Autodesk Fusion 360 part; units mm, degrees
(part 2 of 2)
sketch "Sketch1 (1)" plane through (0, 0, 0) normal (0, 0, -1) x (1, 0, 0) in component "volleyball"
  arc A0 (83.3961, -53.0936) -> (83.8923, -52.463) centre (16.2304, 0.2686) ccw
  spline S0 degree 3 poles (83.1659, -53.382) (83.2447, -53.2843) (83.3214, -53.1882) (83.3961, -53.0936) knots 0.976391 0.976391 0.976391 0.976391 1 1 1 1
  arc A1 (-51.0592, -52.9372) -> (83.1659, -53.382) centre (16.2304, 0.2686) ccw
  spline S1 degree 3 poles (-51.3776, -52.5454) (-51.2718, -52.6763) (-51.1657, -52.8069) (-51.0592, -52.9372) knots 0 0 0 0 0.021256 0.021256 0.021256 0.021256
  line L0 (-51.3776, -52.5454) -> (-52.9378, -50.6056)
  line L1 (-52.9378, -50.6056) -> (-52.8595, -50.5775)
  arc A2 (-55.8686, -46.2124) -> (-52.8595, -50.5775) centre (16.2304, 0.2686) ccw
  line L2 (-55.8686, -46.2124) -> (-55.8897, -46.22)
  line L3 (-55.8897, -46.22) -> (-57.1969, -44.238)
  spline S2 degree 3 poles (-62.1595, -34.5706) (-60.5198, -38.328) (-58.7655, -41.7837) (-57.1969, -44.238) knots 0.562392 0.562392 0.562392 0.562392 1 1 1 1
  arc A3 (-63.9062, -30.3398) -> (-62.1595, -34.5706) centre (16.2304, 0.2686) ccw
  spline S3 degree 3 poles (-67.2754, -20.0749) (-66.4965, -23.1736) (-65.2961, -26.7754) (-63.9062, -30.3398) knots 0 0 0 0 0.401537 0.401537 0.401537 0.401537
  spline S4 degree 3 poles (-68.058, -15.6752) (-68.2174, -16.4999) (-67.8619, -17.7657) (-67.2754, -20.0749) knots 0.565386 0.565386 0.565386 0.565386 1 1 1 1
  arc A4 (-69.0247, -9.2348) -> (-68.058, -15.6752) centre (16.2304, 0.2686) ccw
  spline S5 degree 3 poles (-69.6369, 4.7629) (-69.9364, -0.9646) (-69.6045, -7.9217) (-69.0247, -9.2348) knots 0 0 0 0 0.88772 0.88772 0.88772 0.88772
  spline S6 degree 3 poles (-68.8618, 11.1337) (-69.2237, 11.4542) (-69.4071, 9.4617) (-69.6369, 4.7629) knots 0.394417 0.394417 0.394417 0.394417 1 1 1 1
  arc A5 (-64.9144, 28.094) -> (-68.8618, 11.1337) centre (16.2304, 0.2686) ccw
  spline S7 degree 3 poles (-62.9742, 34.0285) (-64.2565, 31.0558) (-64.713, 29.8758) (-64.9144, 28.094) knots 0 0 0 0 0.691116 0.691116 0.691116 0.691116
  spline S8 degree 3 poles (-45.01, 60.7639) (-52.3475, 53.3421) (-58.715, 43.8962) (-62.9742, 34.0285) knots 0 0 0 0 1 1 1 1
  spline S9 degree 3 poles (-33.6664, 70.3786) (-33.9616, 70.7159) (-41.2147, 64.5592) (-45.01, 60.7639) knots 0 0 0 0 1 1 1 1
  spline S10 degree 3 poles (-33.7771, 69.9679) (-33.6841, 70.2186) (-33.6421, 70.3665) (-33.6664, 70.3786) knots 0.712651 0.712651 0.712651 0.712651 1 1 1 1
  arc A6 (-23.4578, 76.3185) -> (-33.7771, 69.9679) centre (16.2304, 0.2686) ccw
  spline S11 degree 3 poles (-18.6119, 79.1077) (-21.4959, 77.8353) (-22.4841, 77.3971) (-23.4578, 76.3185) knots 0 0 0 0 0.670505 0.670505 0.670505 0.670505
  spline S12 degree 3 poles (8.1657, 86.15) (-0.9429, 85.2222) (-10.2202, 82.7764) (-18.6119, 79.1077) knots 0 0 0 0 1 1 1 1
  spline S13 degree 3 poles (13.4592, 86.007) (13.6596, 86.7737) (12.1492, 86.5306) (8.1657, 86.15) knots 0.398323 0.398323 0.398323 0.398323 1 1 1 1
  arc A7 (21.8306, 85.8687) -> (13.4592, 86.007) centre (16.2304, 0.2686) ccw
  spline S14 degree 3 poles (25.8347, 85.9813) (23.1616, 86.2075) (21.822, 86.183) (21.8306, 85.8687) knots 0 0 0 0 0.487624 0.487624 0.487624 0.487624
  spline S15 degree 3 poles (52.2328, 78.6016) (44.3893, 82.2282) (33.4674, 85.2644) (25.8347, 85.9813) knots 0 0 0 0 1 1 1 1
  spline S16 degree 3 poles (91.8721, 41.3238) (82.7214, 57.8121) (68.7633, 70.969) (52.2328, 78.6016) knots 0 0 0 0 1 1 1 1
  spline S17 degree 3 poles (93.3059, 38.4985) (93.3902, 38.4985) (92.7577, 39.7636) (91.8721, 41.3238) knots 0 0 0 0 1 1 1 1
  spline S18 degree 3 poles (92.6292, 39.281) (93.0311, 38.7947) (93.287, 38.4985) (93.3059, 38.4985) knots 0.551981 0.551981 0.551981 0.551981 1 1 1 1
  arc A8 (101.1344, 12.5184) -> (92.6292, 39.281) centre (16.2304, 0.2686) ccw
  spline S19 degree 3 poles (102.2458, 0.5459) (102.2458, 5.3459) (101.8846, 9.2629) (101.1344, 12.5184) knots 0 0 0 0 0.689854 0.689854 0.689854 0.689854
  spline S20 degree 3 poles (98.7879, -23.4906) (100.7699, -16.9544) (102.2458, -6.7494) (102.2458, 0.5459) knots 0 0 0 0 1 1 1 1
  spline S21 degree 3 poles (97.7675, -26.3857) (97.9614, -25.9701) (98.3902, -24.7924) (98.7879, -23.4906) knots 0.142524 0.142524 0.142524 0.142524 1 1 1 1
  arc A9 (94.2462, -35.4005) -> (97.7675, -26.3857) centre (16.2304, 0.2686) ccw
  line L4 (94.2462, -35.4005) -> (94.318, -35.6776)
  line L5 (94.318, -35.6776) -> (92.5468, -39.009)
  spline S22 degree 3 poles (91.7936, -40.3388) (92.0288, -39.9459) (92.2777, -39.5051) (92.5468, -39.009) knots 0.80059 0.80059 0.80059 0.80059 1 1 1 1
  arc A10 (85.3416, -50.5487) -> (91.7936, -40.3388) centre (16.2304, 0.2686) ccw
  line L6 (85.3416, -50.5487) -> (85.4202, -50.5213)
  line L7 (85.4202, -50.5213) -> (83.8923, -52.463)
  spline S23 degree 3 poles (15.4189, -90.4979) (12.72, -90.4558) (8.9248, -90.2449) (6.9428, -90.0762) knots 0 0 0 0 1 1 1 1
  spline S24 degree 3 poles (102.6253, -27.8341) (90.354, -65.4493) (54.8473, -90.9196) (15.4189, -90.4979) knots 0 0 0 0 1 1 1 1
  spline S25 degree 3 poles (98.2397, 39.9744) (108.5291, 18.6788) (110.0472, -5.1048) (102.6253, -27.8341) knots 0 0 0 0 1 1 1 1
  spline S26 degree 3 poles (29.9252, 90.5778) (59.4438, 86.0656) (85.2093, 66.9629) (98.2397, 39.9744) knots 0 0 0 0 1 1 1 1
  spline S27 degree 3 poles (-48.0883, 64.8544) (-27.594, 85.3066) (1.5451, 94.9212) (29.9252, 90.5778) knots 0 0 0 0 1 1 1 1
  spline S28 degree 3 poles (-73.137, 17.8354) (-69.7213, 35.5888) (-61.0344, 51.9084) (-48.0883, 64.8544) knots 0 0 0 0 1 1 1 1
  spline S29 degree 3 poles (-48.0462, -63.7625) (-69.5526, -42.2982) (-78.872, -11.9784) (-73.137, 17.8354) knots 0 0 0 0 1 1 1 1
  spline S30 degree 3 poles (6.9428, -90.0762) (-13.5515, -87.9678) (-33.2869, -78.5218) (-48.0462, -63.7625) knots 0 0 0 0 1 1 1 1
  line L8 (-29.2215, 67.0521) -> (-27.2782, 62.1333)
  line L9 (16.0482, 23.5133) -> (16.9632, 18.2905)
  spline S31 degree 5 poles (-29.2215, 67.0521) (-27.2169, 67.844) (-23.1769, 69.2849) (-17.024, 71.0173) (-8.6346, 72.4691) (2.1466, 72.8543) (13.1771, 71.8135) (24.3659, 69.3547) (35.5625, 65.493) (46.5368, 60.2511) (56.9839, 53.666) (66.561, 45.8033) (74.916, 36.7693) (81.7202, 26.725) (86.6971, 15.8966) (89.658, 4.5944) (90.5182, -6.7944) (89.2793, -17.8574) (86.0193, -28.199) (80.8797, -37.4875) (74.0534, -45.4973) (65.7727, -52.1602) (56.2994, -57.5184) (45.9154, -61.6662) (34.9127, -64.694) (23.5847, -66.6367) (12.2152, -67.406) (1.0725, -66.7803) (-9.5904, -64.493) (-19.5366, -60.2966) (-28.5457, -54.0387) (-36.4147, -45.7289) (-42.9583, -35.6201) (-48.0121, -24.156) (-51.436, -11.9035) (-53.1176, 0.5089) (-52.9751, 12.4565) (-50.9619, 23.3791) (-47.0678, 32.8512) (-41.3393, 40.5784) (-33.9011, 46.3842) (-24.9773, 50.2007) (-14.9142, 52.0569) (-4.1988, 52.0687) (6.6205, 50.4191) (17.0078, 47.3391) (26.5192, 43.0888) (34.8719, 37.9381) (42.0397, 32.1478) (48.183, 25.9467) (53.5283, 19.5052) (58.2702, 12.9137) (62.4513, 6.1495) (65.8917, -0.9205) (68.2704, -8.4102) (69.1824, -16.3147) (68.2025, -24.3802) (64.9542, -32.0442) (59.2196, -38.632) (51.0385, -43.5102) (40.8208, -46.2648) (29.4276, -46.8464) (17.9319, -45.4469) (7.4086, -42.3984) (-1.2948, -38.0598) (-7.7599, -32.7173) (-12.2637, -26.4576) (-15.508, -19.2522) (-18.2296, -11.086) (-20.8924, -2.0588) (-23.2444, 7.473) (-24.4506, 16.9184) (-23.5181, 25.5534) (-19.6156, 32.5976) (-12.4698, 37.3008) (-2.6303, 39.0279) (8.8236, 37.3599) (20.5053, 32.1955) (30.9661, 23.8455) (38.9401, 13.1478) (43.562, 1.5221) (44.366, -9.3682) (41.3136, -17.9198) (34.8027, -22.886) (25.7036, -23.7254) (15.3263, -20.7758) (5.2068, -14.9206) (-3.0832, -7.3376) (-8.1196, 0.7654) (-8.8494, 8.4547) (-4.9032, 14.8085) (1.8086, 18.9695) (8.6695, 21.5297) (13.7833, 22.9537) (16.0482, 23.5133) knots 0 0 0 0 0 0 0.01111111 0.02222222 0.03333333 0.04444444 0.05555556 0.06666667 0.07777778 0.08888889 0.1 0.11111111 0.12222222 0.13333333 0.14444444 0.15555556 0.16666667 0.17777778 0.18888889 0.2 0.21111111 0.22222222 0.23333333 0.24444444 0.25555556 0.26666667 0.27777778 0.28888889 0.3 0.31111111 0.32222222 0.33333333 0.34444444 0.35555556 0.36666667 0.37777778 0.38888889 0.4 0.41111111 0.42222222 0.43333333 0.44444444 0.45555556 0.46666667 0.47777778 0.48888889 0.5 0.51111111 0.52222222 0.53333333 0.54444444 0.55555556 0.56666667 0.57777778 0.58888889 0.6 0.61111111 0.62222222 0.63333333 0.64444444 0.65555556 0.66666667 0.67777778 0.68888889 0.7 0.71111111 0.72222222 0.73333333 0.74444444 0.75555556 0.76666667 0.77777778 0.78888889 0.8 0.81111111 0.82222222 0.83333333 0.84444444 0.85555556 0.86666667 0.87777778 0.88888889 0.9 0.91111111 0.92222222 0.93333333 0.94444444 0.95555556 0.96666667 0.97777778 0.98888889 0.99681722 0.99681722 0.99681722 0.99681722 0.99681722 0.99681722
  line L10 (-40.3037, 9.5917) -> (72.4001, 37.4349)
  spline S32 degree 3 poles (-27.2782, 62.1333) (-18.4995, 65.6015) (-9.3846, 67.2981) (0.1399, 67.2455) (8.5571, 67.199) (17.3131, 65.7722) (26.0845, 62.9636) (36.0331, 59.778) (45.989, 54.7984) (54.769, 48.2524) (62.7383, 42.3109) (69.6918, 35.0766) (74.8036, 27.0265) (79.4688, 19.6797) (82.5941, 11.6494) (83.9381, 3.5764) (85.3228, -4.7407) (84.8198, -13.0634) (82.596, -20.5598) (80.5257, -27.5383) (76.9917, -33.7755) (72.2591, -39.0259) (66.6139, -45.2888) (59.2098, -50.2) (50.6864, -53.8542) (42.3154, -57.443) (32.8909, -59.8628) (23.4649, -61.0282) (14.7481, -62.1058) (6.0747, -62.0747) (-1.8615, -60.4969) (-9.0504, -59.0676) (-15.6425, -56.3638) (-21.5007, -52.1365) (-26.4018, -48.5999) (-30.8117, -43.9659) (-34.5628, -38.373) (-39.0655, -31.6592) (-42.5898, -23.5744) (-44.8022, -15.1377) (-46.9488, -6.9522) (-47.8539, 1.5218) (-47.4299, 9.1977) (-47.0493, 16.0893) (-45.6019, 22.3071) (-43.227, 27.4201) (-39.6512, 35.1184) (-34.0621, 40.3844) (-26.5437, 43.457) (-21.5214, 45.5096) (-15.6054, 46.5425) (-9.3298, 46.5555) (-2.0953, 46.5706) (5.5514, 45.2302) (12.5806, 42.9133) (18.6007, 40.929) (24.1457, 38.2477) (28.9794, 35.1628) (36.1545, 30.5835) (41.8183, 25.133) (46.6569, 19.3732) (50.2237, 15.1273) (53.3846, 10.712) (56.066, 6.2493) (59.3085, 0.8525) (61.8032, -4.6535) (62.8659, -10.2934) (63.7446, -14.9565) (63.6229, -19.7362) (62.1653, -24.1034) (60.6037, -28.7824) (57.542, -32.9474) (52.6166, -36.0009) (49.3573, -38.0216) (45.2466, -39.5359) (40.5565, -40.3584) (34.6839, -41.3881) (27.9526, -41.311) (21.5983, -40.2819) (16.0907, -39.3898) (10.9025, -37.8049) (6.6508, -35.8242) (3.1261, -34.1821) (0.2593, -32.2894) (-2.015, -30.231) (-4.9267, -27.5958) (-6.953, -24.6635) (-8.7185, -21.0479) (-10.3736, -17.6583) (-11.7932, -13.6467) (-13.1932, -9.1928) (-14.6123, -4.6781) (-16.0267, 0.2651) (-17.0929, 5.1134) (-18.0425, 9.4313) (-18.6693, 13.6692) (-18.6274, 17.3333) (-18.5919, 20.4409) (-18.0776, 23.0936) (-17.1057, 25.2016) (-16.1093, 27.3626) (-14.6665, 29.0337) (-12.5073, 30.3612) (-10.4073, 31.6522) (-7.5777, 32.5707) (-4.158, 32.8224) (0.0973, 33.1357) (5.2219, 32.3805) (10.364, 30.3987) (15.4301, 28.4461) (20.4894, 25.3085) (24.7965, 21.3017) (29.0165, 17.376) (32.5094, 12.6142) (34.8375, 7.7563) (36.9738, 3.2986) (38.1157, -1.218) (38.2618, -5.0224) (38.3753, -7.9764) (37.8974, -10.4715) (37.0731, -12.3156) (36.3271, -13.9845) (35.3457, -15.1395) (34.098, -15.9875) (32.8173, -16.8578) (31.1779, -17.4316) (29.0496, -17.5874) (26.5047, -17.7737) (23.2947, -17.2973) (19.8988, -16.1263) (15.4038, -14.5763) (10.6242, -11.8298) (6.7111, -8.6153) (3.4575, -5.9425) (0.8189, -2.9563) (-0.7593, -0.2828) (-1.8663, 1.5924) (-2.4457, 3.2846) (-2.6071, 4.6508) (-2.7539, 5.8925) (-2.6132, 6.8669) (-2.1737, 7.8865) (-1.7195, 8.9403) (-0.8855, 10.098) (0.6443, 11.3581) (2.762, 13.1024) (6.214, 14.9489) (11.0293, 16.5691) (12.8232, 17.1727) (14.8025, 17.7481) (16.9632, 18.2905) knots 0 0 0 0 0.03125 0.03125 0.03125 0.05886725 0.05886725 0.05886725 0.09019107 0.09019107 0.09019107 0.1186226 0.1186226 0.1186226 0.14457021 0.14457021 0.14457021 0.17130239 0.17130239 0.17130239 0.19618794 0.19618794 0.19618794 0.22587269 0.22587269 0.22587269 0.25502621 0.25502621 0.25502621 0.28198592 0.28198592 0.28198592 0.30640698 0.30640698 0.30640698 0.32683821 0.32683821 0.32683821 0.35136381 0.35136381 0.35136381 0.37515917 0.37515917 0.37515917 0.39652337 0.39652337 0.39652337 0.4286896 0.4286896 0.4286896 0.45017647 0.45017647 0.45017647 0.4749466 0.4749466 0.4749466 0.49616077 0.49616077 0.49616077 0.52765072 0.52765072 0.52765072 0.55086359 0.55086359 0.55086359 0.57893462 0.57893462 0.57893462 0.60214367 0.60214367 0.60214367 0.62700969 0.62700969 0.62700969 0.64346457 0.64346457 0.64346457 0.66406799 0.66406799 0.66406799 0.68192622 0.68192622 0.68192622 0.69673125 0.69673125 0.69673125 0.71568555 0.71568555 0.71568555 0.7334552 0.7334552 0.7334552 0.7514676 0.7514676 0.7514676 0.76750937 0.76750937 0.76750937 0.78111437 0.78111437 0.78111437 0.79506116 0.79506116 0.79506116 0.80862578 0.80862578 0.80862578 0.82550479 0.82550479 0.82550479 0.84213398 0.84213398 0.84213398 0.85842643 0.85842643 0.85842643 0.87337664 0.87337664 0.87337664 0.8849853 0.8849853 0.8849853 0.8954918 0.8954918 0.8954918 0.90627553 0.90627553 0.90627553 0.91917069 0.91917069 0.91917069 0.93623974 0.93623974 0.93623974 0.95043241 0.95043241 0.95043241 0.96038732 0.96038732 0.96038732 0.96943543 0.96943543 0.96943543 0.97878732 0.97878732 0.97878732 0.99173272 0.99173272 0.99173272 0.9965555 0.9965555 0.9965555 0.9965555
  point P0 (30.5171, 67.0521)
  point P1 (84.6365, 19.7296)
  point P2 (79.7844, -38.1222)
  point P3 (27.9044, -65.7418)
  point P4 (-29.2215, -52.6785)
  point P5 (-52.3416, 13.7578)
  point P6 (-25.0953, 49.5886)
  point P7 (28.2776, 41.7506)
  point P8 (57.0169, 14.5042)
  point P9 (68.6799, -14.6083)
  point P10 (51.4183, -42.6011)
  point P11 (-1.9546, -37.0025)
  point P12 (-19.1235, -7.89)
  point P13 (-19.7557, 30.9267)
  point P14 (29.0241, 24.5825)
  point P15 (36.1156, -20.9533)
  point P16 (-5.4919, -2.6647)
  point P17 (-29.2215, 67.0521)
  constraint coincident P17 L8.start
  constraint midpoint L9.start L10
extrude "Extrude1'''" cut sketch "Sketch1 (1)" against normal blind 15 contours L8 S31 L10 S32 | S31 L10 S32 | S31 L10 S32 | L9 S31 L10 S32 picked at (-14.7988, -9.249) picked at (-22.0722, 15.8634) bodies 2 in component "volleyball"
sketch "Sketch2 (1)" plane through (0, 0, 0) normal (0, 0, -1) x (1, 0, 0) in component "volleyball"
  arc A0 (83.3961, -53.0936) -> (83.8923, -52.463) centre (16.2304, 0.2686) ccw
  spline S0 degree 3 poles (83.1659, -53.382) (83.2447, -53.2843) (83.3214, -53.1882) (83.3961, -53.0936) knots 0.976391 0.976391 0.976391 0.976391 1 1 1 1
  arc A1 (-51.0592, -52.9372) -> (83.1659, -53.382) centre (16.2304, 0.2686) ccw
  spline S1 degree 3 poles (-51.3776, -52.5454) (-51.2718, -52.6763) (-51.1657, -52.8069) (-51.0592, -52.9372) knots 0 0 0 0 0.021256 0.021256 0.021256 0.021256
  line L0 (-51.3776, -52.5454) -> (-52.9378, -50.6056)
  line L1 (-52.9378, -50.6056) -> (-52.8595, -50.5775)
  arc A2 (-55.8686, -46.2124) -> (-52.8595, -50.5775) centre (16.2304, 0.2686) ccw
  line L2 (-55.8686, -46.2124) -> (-55.8897, -46.22)
  line L3 (-55.8897, -46.22) -> (-57.1969, -44.238)
  spline S2 degree 3 poles (-62.1595, -34.5706) (-60.5198, -38.328) (-58.7655, -41.7837) (-57.1969, -44.238) knots 0.562392 0.562392 0.562392 0.562392 1 1 1 1
  arc A3 (-63.9062, -30.3398) -> (-62.1595, -34.5706) centre (16.2304, 0.2686) ccw
  spline S3 degree 3 poles (-67.2754, -20.0749) (-66.4965, -23.1736) (-65.2961, -26.7754) (-63.9062, -30.3398) knots 0 0 0 0 0.401537 0.401537 0.401537 0.401537
  spline S4 degree 3 poles (-68.058, -15.6752) (-68.2174, -16.4999) (-67.8619, -17.7657) (-67.2754, -20.0749) knots 0.565386 0.565386 0.565386 0.565386 1 1 1 1
  arc A4 (-69.0247, -9.2348) -> (-68.058, -15.6752) centre (16.2304, 0.2686) ccw
  spline S5 degree 3 poles (-69.6369, 4.7629) (-69.9364, -0.9646) (-69.6045, -7.9217) (-69.0247, -9.2348) knots 0 0 0 0 0.88772 0.88772 0.88772 0.88772
  spline S6 degree 3 poles (-68.8618, 11.1337) (-69.2237, 11.4542) (-69.4071, 9.4617) (-69.6369, 4.7629) knots 0.394417 0.394417 0.394417 0.394417 1 1 1 1
  arc A5 (-64.9144, 28.094) -> (-68.8618, 11.1337) centre (16.2304, 0.2686) ccw
  spline S7 degree 3 poles (-62.9742, 34.0285) (-64.2565, 31.0558) (-64.713, 29.8758) (-64.9144, 28.094) knots 0 0 0 0 0.691116 0.691116 0.691116 0.691116
  spline S8 degree 3 poles (-45.01, 60.7639) (-52.3475, 53.3421) (-58.715, 43.8962) (-62.9742, 34.0285) knots 0 0 0 0 1 1 1 1
  spline S9 degree 3 poles (-33.6664, 70.3786) (-33.9616, 70.7159) (-41.2147, 64.5592) (-45.01, 60.7639) knots 0 0 0 0 1 1 1 1
  spline S10 degree 3 poles (-33.7771, 69.9679) (-33.6841, 70.2186) (-33.6421, 70.3665) (-33.6664, 70.3786) knots 0.712651 0.712651 0.712651 0.712651 1 1 1 1
  arc A6 (-23.4578, 76.3185) -> (-33.7771, 69.9679) centre (16.2304, 0.2686) ccw
  spline S11 degree 3 poles (-18.6119, 79.1077) (-21.4959, 77.8353) (-22.4841, 77.3971) (-23.4578, 76.3185) knots 0 0 0 0 0.670505 0.670505 0.670505 0.670505
  spline S12 degree 3 poles (8.1657, 86.15) (-0.9429, 85.2222) (-10.2202, 82.7764) (-18.6119, 79.1077) knots 0 0 0 0 1 1 1 1
  spline S13 degree 3 poles (13.4592, 86.007) (13.6596, 86.7737) (12.1492, 86.5306) (8.1657, 86.15) knots 0.398323 0.398323 0.398323 0.398323 1 1 1 1
  arc A7 (21.8306, 85.8687) -> (13.4592, 86.007) centre (16.2304, 0.2686) ccw
  spline S14 degree 3 poles (25.8347, 85.9813) (23.1616, 86.2075) (21.822, 86.183) (21.8306, 85.8687) knots 0 0 0 0 0.487624 0.487624 0.487624 0.487624
  spline S15 degree 3 poles (52.2328, 78.6016) (44.3893, 82.2282) (33.4674, 85.2644) (25.8347, 85.9813) knots 0 0 0 0 1 1 1 1
  spline S16 degree 3 poles (91.8721, 41.3238) (82.7214, 57.8121) (68.7633, 70.969) (52.2328, 78.6016) knots 0 0 0 0 1 1 1 1
  spline S17 degree 3 poles (93.3059, 38.4985) (93.3902, 38.4985) (92.7577, 39.7636) (91.8721, 41.3238) knots 0 0 0 0 1 1 1 1
  spline S18 degree 3 poles (92.6292, 39.281) (93.0311, 38.7947) (93.287, 38.4985) (93.3059, 38.4985) knots 0.551981 0.551981 0.551981 0.551981 1 1 1 1
  arc A8 (101.1344, 12.5184) -> (92.6292, 39.281) centre (16.2304, 0.2686) ccw
  spline S19 degree 3 poles (102.2458, 0.5459) (102.2458, 5.3459) (101.8846, 9.2629) (101.1344, 12.5184) knots 0 0 0 0 0.689854 0.689854 0.689854 0.689854
  spline S20 degree 3 poles (98.7879, -23.4906) (100.7699, -16.9544) (102.2458, -6.7494) (102.2458, 0.5459) knots 0 0 0 0 1 1 1 1
  spline S21 degree 3 poles (97.7675, -26.3857) (97.9614, -25.9701) (98.3902, -24.7924) (98.7879, -23.4906) knots 0.142524 0.142524 0.142524 0.142524 1 1 1 1
  arc A9 (94.2462, -35.4005) -> (97.7675, -26.3857) centre (16.2304, 0.2686) ccw
  line L4 (94.2462, -35.4005) -> (94.318, -35.6776)
  line L5 (94.318, -35.6776) -> (92.5468, -39.009)
  spline S22 degree 3 poles (91.7936, -40.3388) (92.0288, -39.9459) (92.2777, -39.5051) (92.5468, -39.009) knots 0.80059 0.80059 0.80059 0.80059 1 1 1 1
  arc A10 (85.3416, -50.5487) -> (91.7936, -40.3388) centre (16.2304, 0.2686) ccw
  line L6 (85.3416, -50.5487) -> (85.4202, -50.5213)
  line L7 (85.4202, -50.5213) -> (83.8923, -52.463)
  spline S23 degree 3 poles (15.4189, -90.4979) (12.72, -90.4558) (8.9248, -90.2449) (6.9428, -90.0762) knots 0 0 0 0 1 1 1 1
  spline S24 degree 3 poles (102.6253, -27.8341) (90.354, -65.4493) (54.8473, -90.9196) (15.4189, -90.4979) knots 0 0 0 0 1 1 1 1
  spline S25 degree 3 poles (98.2397, 39.9744) (108.5291, 18.6788) (110.0472, -5.1048) (102.6253, -27.8341) knots 0 0 0 0 1 1 1 1
  spline S26 degree 3 poles (29.9252, 90.5778) (59.4438, 86.0656) (85.2093, 66.9629) (98.2397, 39.9744) knots 0 0 0 0 1 1 1 1
  spline S27 degree 3 poles (-48.0883, 64.8544) (-27.594, 85.3066) (1.5451, 94.9212) (29.9252, 90.5778) knots 0 0 0 0 1 1 1 1
  spline S28 degree 3 poles (-73.137, 17.8354) (-69.7213, 35.5888) (-61.0344, 51.9084) (-48.0883, 64.8544) knots 0 0 0 0 1 1 1 1
  spline S29 degree 3 poles (-48.0462, -63.7625) (-69.5526, -42.2982) (-78.872, -11.9784) (-73.137, 17.8354) knots 0 0 0 0 1 1 1 1
  spline S30 degree 3 poles (6.9428, -90.0762) (-13.5515, -87.9678) (-33.2869, -78.5218) (-48.0462, -63.7625) knots 0 0 0 0 1 1 1 1
  line L8 (47.0665, 78.0426) -> (53.3064, 75.2645)
  line L9 (53.3064, 75.2645) -> (60.8616, 92.2344)
  line L10 (60.8616, 92.2344) -> (54.6217, 95.0125)
  line L11 (54.6217, 95.0125) -> (47.0665, 78.0426)
  line L12 (-12.0387, 97.2712) -> (-2.218, 98.7101)
  line L13 (-2.218, 98.7101) -> (0.7475, 78.4698)
  line L14 (0.7475, 78.4698) -> (-9.0733, 77.031)
  line L15 (-9.0733, 77.031) -> (-12.0387, 97.2712)
  constraint perpendicular L8 L9
  constraint parallel L8 L10
  constraint parallel L9 L11
  constraint perpendicular L12 L13
  constraint parallel L12 L14
  constraint parallel L13 L15
extrude "Extrude2'''" cut sketch "Sketch2 (1)" against normal blind 15 contours S15 S16 L8 L9 L11 | S15 S16 S26 L9 L11 | S26 L9 L10 L11 | S12 S27 L13 L15 | S27 L12 L13 L15 | S12 L13 L14 L15 bodies 2 in component "volleyball"
extrude "Extrude11" cut sketch "Sketch2 (1)" against normal blind 15 contours S15 S16 L8 L9 L11 | S15 S16 S26 L9 L11 | S26 L9 L10 L11 | S12 S27 L13 L15 | S27 L12 L13 L15 | S12 L13 L14 L15 bodies 4 in component "base"
sketch "Sketch5" plane through (0, 0, 19) normal (0, 0, -1) x (1, 0, 0) in component "base"
  line L0 (-45.0632, 95.9081) -> (-23.0632, 95.9081)
  line L1 (-23.0632, 95.9081) -> (-23.0632, 117.9081)
  line L2 (-23.0632, 117.9081) -> (-45.0632, 117.9081)
  line L3 (-45.0632, 117.9081) -> (-45.0632, 95.9081)
  line L4 (-38.7298, 95.9081) -> (-27.195, 95.9081)
  line L5 (-27.195, 95.9081) -> (-27.195, 104.1082)
  line L6 (-27.195, 104.1082) -> (-38.7298, 104.1082)
  line L7 (-38.7298, 104.1082) -> (-38.7298, 95.9081)
  constraint horizontal L4
  constraint vertical L5
  constraint horizontal L6
  constraint vertical L7
  constraint coincident L0 L4.start
extrude "Extrude12" cut sketch "Sketch5" against normal blind 55 contours L0 L4 L5 L6 L7 bodies 4 8 in component "base"
extrude "Extrude3''" add 1 faces at (89.9079, -47.5871, 0) along direction (0, 0, -1) blind 2.5 on bodies 2 bodies 2 in component "volleyball"
sketch "Sketch1 (3)" plane through (0, 0, -2.5) normal (0, 0, -1) x (1, 0, 0) in component "main_back"
  line L0 (56.392, 82.1951) -> (54.3421, 77.5909)
  spline S0 degree 3 poles (54.3421, 77.5909) (69.9499, 69.836) (83.1132, 57.106) (91.8721, 41.3238) knots -0.957177 -0.957177 -0.957177 -0.957177 0 0 0 0
  spline S1 degree 3 poles (91.8721, 41.3238) (92.7577, 39.7636) (93.3902, 38.4985) (93.3059, 38.4985) knots -1 -1 -1 -1 0 0 0 0
  spline S2 degree 3 poles (93.3059, 38.4985) (93.287, 38.4985) (93.0311, 38.7947) (92.6292, 39.281) knots -1 -1 -1 -1 -0.551981 -0.551981 -0.551981 -0.551981
  arc A0 (101.1344, 12.5184) -> (92.6292, 39.281) centre (16.2304, 0.2686) ccw
  spline S3 degree 3 poles (101.1344, 12.5184) (101.8846, 9.2629) (102.2458, 5.3459) (102.2458, 0.5459) knots -0.689854 -0.689854 -0.689854 -0.689854 0 0 0 0
  spline S4 degree 3 poles (102.2458, 0.5459) (102.2458, -6.7494) (100.7699, -16.9544) (98.7879, -23.4906) knots -1 -1 -1 -1 0 0 0 0
  spline S5 degree 3 poles (98.7879, -23.4906) (98.3902, -24.7924) (97.9614, -25.9701) (97.7675, -26.3857) knots -1 -1 -1 -1 -0.142524 -0.142524 -0.142524 -0.142524
  arc A1 (94.2462, -35.4005) -> (97.7675, -26.3857) centre (16.2304, 0.2686) ccw
  line L1 (94.2462, -35.4005) -> (94.318, -35.6776)
  line L2 (94.318, -35.6776) -> (92.5468, -39.009)
  spline S6 degree 3 poles (92.5468, -39.009) (92.2777, -39.5051) (92.0288, -39.9459) (91.7936, -40.3388) knots -1 -1 -1 -1 -0.80059 -0.80059 -0.80059 -0.80059
  arc A2 (85.3416, -50.5487) -> (91.7936, -40.3388) centre (16.2304, 0.2686) ccw
  line L3 (85.3416, -50.5487) -> (85.4202, -50.5213)
  line L4 (85.4202, -50.5213) -> (83.8923, -52.463)
  arc A3 (83.3961, -53.0936) -> (83.8923, -52.463) centre (16.2304, 0.2686) ccw
  spline S7 degree 3 poles (83.3961, -53.0936) (83.3214, -53.1882) (83.2447, -53.2843) (83.1659, -53.382) knots -1 -1 -1 -1 -0.976391 -0.976391 -0.976391 -0.976391
  arc A4 (-51.0592, -52.9372) -> (83.1659, -53.382) centre (16.2304, 0.2686) ccw
  spline S8 degree 3 poles (-51.0592, -52.9372) (-51.1657, -52.8069) (-51.2718, -52.6763) (-51.3776, -52.5454) knots -0.021256 -0.021256 -0.021256 -0.021256 0 0 0 0
  line L5 (-51.3776, -52.5454) -> (-52.9378, -50.6056)
  line L6 (-52.9378, -50.6056) -> (-52.8595, -50.5775)
  arc A5 (-55.8686, -46.2124) -> (-52.8595, -50.5775) centre (16.2304, 0.2686) ccw
  line L7 (-55.8686, -46.2124) -> (-55.8897, -46.22)
  line L8 (-55.8897, -46.22) -> (-57.1969, -44.238)
  spline S9 degree 3 poles (-57.1969, -44.238) (-58.7655, -41.7837) (-60.5198, -38.328) (-62.1595, -34.5706) knots -1 -1 -1 -1 -0.562392 -0.562392 -0.562392 -0.562392
  arc A6 (-63.9062, -30.3398) -> (-62.1595, -34.5706) centre (16.2304, 0.2686) ccw
  spline S10 degree 3 poles (-63.9062, -30.3398) (-65.2961, -26.7754) (-66.4965, -23.1736) (-67.2754, -20.0749) knots -0.401537 -0.401537 -0.401537 -0.401537 0 0 0 0
  spline S11 degree 3 poles (-67.2754, -20.0749) (-67.8619, -17.7657) (-68.2174, -16.4999) (-68.058, -15.6752) knots -1 -1 -1 -1 -0.565386 -0.565386 -0.565386 -0.565386
  arc A7 (-69.0247, -9.2348) -> (-68.058, -15.6752) centre (16.2304, 0.2686) ccw
  spline S12 degree 3 poles (-69.0247, -9.2348) (-69.6045, -7.9217) (-69.9364, -0.9646) (-69.6369, 4.7629) knots -0.88772 -0.88772 -0.88772 -0.88772 0 0 0 0
  spline S13 degree 3 poles (-69.6369, 4.7629) (-69.4071, 9.4617) (-69.2237, 11.4542) (-68.8618, 11.1337) knots -1 -1 -1 -1 -0.394417 -0.394417 -0.394417 -0.394417
  arc A8 (-64.9144, 28.094) -> (-68.8618, 11.1337) centre (16.2304, 0.2686) ccw
  spline S14 degree 3 poles (-64.9144, 28.094) (-64.713, 29.8758) (-64.2565, 31.0558) (-62.9742, 34.0285) knots -0.691116 -0.691116 -0.691116 -0.691116 0 0 0 0
  spline S15 degree 3 poles (-62.9742, 34.0285) (-58.715, 43.8962) (-52.3475, 53.3421) (-45.01, 60.7639) knots -1 -1 -1 -1 0 0 0 0
  spline S16 degree 3 poles (-45.01, 60.7639) (-41.2147, 64.5592) (-33.9616, 70.7159) (-33.6664, 70.3786) knots -1 -1 -1 -1 0 0 0 0
  spline S17 degree 3 poles (-33.6664, 70.3786) (-33.6421, 70.3665) (-33.6841, 70.2186) (-33.7771, 69.9679) knots -1 -1 -1 -1 -0.712651 -0.712651 -0.712651 -0.712651
  arc A9 (-23.4578, 76.3185) -> (-33.7771, 69.9679) centre (16.2304, 0.2686) ccw
  spline S18 degree 3 poles (-23.4578, 76.3185) (-22.4841, 77.3971) (-21.4959, 77.8353) (-18.6119, 79.1077) knots -0.670505 -0.670505 -0.670505 -0.670505 0 0 0 0
  spline S19 degree 3 poles (-18.6119, 79.1077) (-15.7814, 80.3451) (-12.8502, 81.4434) (-9.8586, 82.3913) knots -1 -1 -1 -1 -0.662705 -0.662705 -0.662705 -0.662705
  line L9 (-9.8586, 82.3913) -> (-10.6034, 87.4747)
  spline S20 degree 3 poles (-10.6034, 87.4747) (-24.5459, 83.1294) (-37.4761, 75.4448) (-48.0883, 64.8544) knots -0.517814 -0.517814 -0.517814 -0.517814 0 0 0 0
  spline S21 degree 3 poles (-48.0883, 64.8544) (-61.0344, 51.9084) (-69.7213, 35.5888) (-73.137, 17.8354) knots -1 -1 -1 -1 0 0 0 0
  spline S22 degree 3 poles (-73.137, 17.8354) (-78.872, -11.9784) (-69.5526, -42.2982) (-48.0462, -63.7625) knots -1 -1 -1 -1 0 0 0 0
  spline S23 degree 3 poles (-48.0462, -63.7625) (-33.2869, -78.5218) (-13.5515, -87.9678) (6.9428, -90.0762) knots -1 -1 -1 -1 0 0 0 0
  spline S24 degree 3 poles (6.9428, -90.0762) (8.9248, -90.2449) (12.72, -90.4558) (15.4189, -90.4979) knots -1 -1 -1 -1 0 0 0 0
  spline S25 degree 3 poles (15.4189, -90.4979) (54.8473, -90.9196) (90.354, -65.4493) (102.6253, -27.8341) knots -1 -1 -1 -1 0 0 0 0
  spline S26 degree 3 poles (102.6253, -27.8341) (110.0472, -5.1048) (108.5291, 18.6788) (98.2397, 39.9744) knots -1 -1 -1 -1 0 0 0 0
  spline S27 degree 3 poles (98.2397, 39.9744) (89.3089, 58.4719) (74.3957, 73.265) (56.392, 82.1951) knots -1 -1 -1 -1 -0.314615 -0.314615 -0.314615 -0.314615
combine "Combine1" operation add target body 9 tool bodies 8 4 in component "base"
component "volleyball" placed x (1, 0, 0) y (0, 1, 0) z (0, 0, 1) at (0, 0, 0)
component "top" placed x (1, 0, 0) y (0, 1, 0) z (0, 0, 1) at (0, 0, 0)
component "base" placed x (1, 0, 0) y (0, 1, 0) z (0, 0, 1) at (0, 0, 0)
component "main_back" placed x (1, 0, 0) y (0, 1, 0) z (0, 0, 1) at (0, 0, 0)
named bodies: "volleyball", "ring", "ir_remote", "power_supply", "base_housing"
